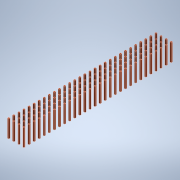
# Autodesk Inventor part: PCIshortpins
Saved by Autodesk Inventor 2022 (Build 260153000, 153)
## iProperties
Created: 2021-10-08
Part Number: PCIshortpins
Material: Copper
Document SubType Name: Modeling
Designer: Bowen O'Steen
Density: 8.94 g/cm^3
Appearance: Copper - Satin
Author: Bowen O'Steen
Autodesk Inventor part; units mm, degrees
ref_plane "YZ Plane" through (0, 0, 0) normal (1, 0, 0) x (0, 1, 0)
ref_plane "XZ Plane" through (0, 0, 0) normal (0, 1, 0) x (-1, 0, 0)
ref_plane "XY Plane" through (0, 0, 0) normal (0, 0, 1) x (1, 0, 0)
sketch "Sketch1" plane through (0, 0, 0) normal (0, 1, 0) x (-1, 0, 0)
  line L0 (0.25, 0.25) -> (-0.25, 0.25)
  line L1 (-0.25, 0.25) -> (-0.25, -0.25)
  line L2 (-0.25, -0.25) -> (0.25, -0.25)
  line L3 (0.25, -0.25) -> (0.25, 0.25)
  point P0 (0, 0)
  point P1 (0.25, 0)
  point P2 (0, -0.25)
  dimension "d0" = 0.5
  dimension "d1" = 0.5
  constraints: 8 end point, 2 midpoint, 2 parallel, 1 horizontal, 1 horizontal alignment, 1 perpendicular, 1 vertical alignment
  measures "d0" distance of L2.end L0.start
  measures "d1" distance of L1.end L2.end
extrude "Extrusion1" add sketch "Sketch1" along normal blind 6.88
pattern_linear "Rectangular Pattern1" count 30 spacing 2 along (0, 0, 1) count 4 spacing 2 along (1, 0, 0) of "Extrusion1"
equation "\"d1\" = d0"
body "Solid1"
